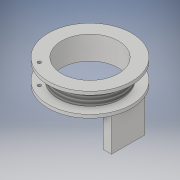
# Autodesk Inventor part: Ttube1
Saved by Autodesk Inventor 2017 (Build 210142000, 142)
## iProperties
Created: 2017-06-28
Part Number: Ttube1
Material: Generic
Document SubType Name: Modeling
Designer: husseinz
Density: 1 g/cm^3
Appearance: Default
Author: husseinz
Autodesk Inventor part; units mm, degrees
ref_plane "YZ Plane" through (0, 0, 0) normal (1, 0, 0) x (0, 1, 0)
ref_plane "XZ Plane" through (0, 0, 0) normal (0, 1, 0) x (-1, 0, 0)
ref_plane "XY Plane" through (0, 0, 0) normal (0, 0, 1) x (1, 0, 0)
sketch "Sketch1" plane through (0, 0, 0) normal (0, 1, 0) x (-1, 0, 0)
  circle A0 centre (0, 0) radius 12.5
  dimension "d0" = 25
  constraints: 1 centre point, 1 coincident
  measures "d0" diameter of A0
extrude "Extrusion1" add sketch "Sketch1" along normal blind 1
sketch "Sketch2" plane through (0, 1, 0) normal (0, 1, 0) x (1, 0, 0)
  circle A0 centre (0, 0) radius 9.5
  dimension "d3" = 19
  constraints: 1 centre point, 1 coincident
  measures "d3" diameter of A0
extrude "Extrusion2" add sketch "Sketch2" along normal blind 5
sketch "Sketch3" plane through (0, 6, 0) normal (0, 1, 0) x (1, 0, 0)
  circle A0 centre (0, 0) radius 12.5
  dimension "d6" = 25
  constraints: 1 centre point, 1 coincident
  measures "d6" diameter of A0
extrude "Extrusion3" add sketch "Sketch3" along normal blind 1
hole "Hole1" at (-6.2494, 7, 8.9167) direction (0, -1, 0) diameter 1 depth 7
sketch "Sketch4" plane through (0, 7, 0) normal (0, 1, 0) x (1, 0, 0)
  circle A0 centre (0, 0) radius 8.5
  dimension "d18" = 17
  constraints: 1 centre point, 1 coincident
  measures "d18" diameter of A0
extrude "Extrusion4" cut sketch "Sketch4" against normal blind 7
thread "Thread1" size "4-24" class "2B" standard "Inch Tapping Threads" full length
sketch "Sketch5" plane through (0, 0, 0) normal (0, -1, 0) x (1, 0, 0)
  line L0 (11.3779, 4.9373) -> (8.8779, 4.9373)
  line L1 (8.8779, 4.9373) -> (8.8779, -5.0627)
  line L2 (8.8779, -5.0627) -> (11.3779, -5.0627)
  line L3 (11.3779, -5.0627) -> (11.3779, 4.9373)
  point P0 (0, 0)
  dimension "d23" = 10
  dimension "d24" = 2.5
  constraints: 8 end point, 2 parallel, 1 horizontal, 1 perpendicular
  measures "d23" distance of L2.end L0.start
  measures "d24" distance of L0.start L0.end
extrude "Extrusion5" add sketch "Sketch5" along normal blind 10
body "Solid1"
